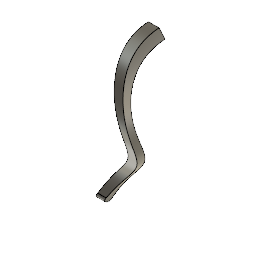
6.5 circular pattern (Autodesk Fusion 360 design; units mm, degrees)
Autodesk Fusion 360 part; units mm, degrees
sketch "Sketch1" plane through (0, 0, 0) normal (1, 0, 0) x (0, 1, 0)
  spline S0 degree 5 poles (0, 0) (-1.5461, -0.056) (-4.5103, -0.2863) (-8.5728, -0.9868) (-13.2055, -2.6049) (-17.6093, -5.6119) (-20.5447, -9.3915) (-21.9764, -13.7078) (-21.9581, -18.3281) (-20.7021, -23.054) (-18.5832, -27.735) (-16.0525, -32.2598) (-13.5801, -36.5535) (-11.5892, -40.5752) (-10.3932, -44.316) (-10.1254, -47.8001) (-10.6672, -50.4131) (-11.4827, -52.2914) (-12.2041, -53.5097) (-12.6092, -54.1104) knots 0 0 0 0 0 0 0.066667 0.133333 0.2 0.266667 0.333333 0.4 0.466667 0.533333 0.6 0.666667 0.733333 0.8 0.866667 0.933333 1 1 1 1 1 1
  line L0 (10.2739, 0.3719) -> (-10.2739, -0.3719)
  spline S1 degree 3 poles (0.1, -2.7622) (-6.0917, -2.9863) (-10.7245, -4.4824) (-13.8238, -6.6593) (-16.4227, -8.4848) (-17.9499, -10.7212) (-18.6267, -13.1732) (-19.304, -15.6268) (-19.1099, -18.3726) (-18.1871, -21.3366) (-17.1185, -24.7688) (-15.0764, -28.4198) (-13.0449, -32.0268) (-10.8363, -35.9482) (-8.7042, -39.8469) (-7.8006, -43.7909) (-7.1465, -46.6457) (-7.1496, -49.5409) (-7.9606, -52.2548) (-8.3548, -53.5742) (-8.9304, -54.8446) (-9.6679, -56.0549) knots 0 0 0 0 0.16767 0.16767 0.16767 0.30827 0.30827 0.30827 0.448963 0.448963 0.448963 0.611881 0.611881 0.611881 0.789001 0.789001 0.789001 0.917212 0.917212 0.917212 0.979548 0.979548 0.979548 0.979548
  line L1 (-12.2892, -55.9) -> (-11.545, -56.4354)
  line L2 (0, 0) -> (0.1, -2.7622)
  arc A0 (-12.6092, -54.1104) -> (-12.2892, -55.9) centre (-11.5269, -54.8403) ccw
  arc A1 (-11.545, -56.4354) -> (-9.6679, -56.0549) centre (-10.7827, -55.3757) ccw
  point P0 (-11.7402, -40.6199)
  dimension "d2" = 1.3054
  constraint coincident S0.start L2.start
  constraint midpoint S0.start L0
  constraint tangent S0 A0
  constraint tangent L1 A0
  constraint tangent L1 A1
  constraint tangent S1 A1
  constraint equal A0 A1
  measures "d2" radius of A0
sketch "Sketch2" plane through (0, 0, 0) normal (0, 1, 0) x (1, 0, 0)
  spline S0 degree 5 poles (-12.1026, -4.473) (-11.4157, -3.9229) (-10.0727, -2.8011) (-8.1507, -1.0537) (-5.7739, 1.4062) (-3.1241, 4.6972) (-0.8218, 8.197) (1.0858, 11.8869) (2.526, 15.7315) (3.3928, 19.6719) (3.574, 23.6369) (2.9838, 27.5566) (1.5945, 31.3748) (-0.5288, 35.0626) (-3.1973, 38.6306) (-6.1455, 42.1158) (-9.0701, 45.5713) (-11.6717, 49.0549) (-13.6924, 52.6195) (-14.9643, 56.3) (-15.3996, 60.1153) (-15.05, 63.2818) (-14.3933, 65.7216) (-13.7809, 67.3768) (-13.431, 68.2116) knots 0 0 0 0 0 0 0.05 0.1 0.15 0.2 0.25 0.3 0.35 0.4 0.45 0.5 0.55 0.6 0.65 0.7 0.75 0.8 0.85 0.9 0.95 1 1 1 1 1 1
  spline S1 degree 3 poles (-10.1736, -6.8817) (-5.8254, -3.3995) (-2.1215, 0.602) (0.7843, 5.1235) (3.2088, 8.8961) (5.0948, 13.0413) (5.978, 17.4473) (6.6428, 20.764) (6.6923, 24.2313) (5.9419, 27.5965) (5.2452, 30.7205) (3.8541, 33.7189) (2.0777, 36.4763) (-0.3869, 40.3021) (-3.5439, 43.7195) (-6.1481, 46.9634) (-8.2297, 49.5562) (-9.9166, 52.025) (-10.9152, 54.4302) (-12.1481, 57.3997) (-12.4388, 60.2799) (-11.7039, 63.5633) (-11.4557, 64.6723) (-11.0858, 65.8238) (-10.585, 67.0188) knots 0 0 0 0 0.179562 0.179562 0.179562 0.329386 0.329386 0.329386 0.442169 0.442169 0.442169 0.546866 0.546866 0.546866 0.692126 0.692126 0.692126 0.808235 0.808235 0.808235 0.951586 0.951586 0.951586 1 1 1 1
  line L0 (-10.1736, -6.8817) -> (-12.1026, -4.473)
  line L1 (-10.585, 67.0188) -> (-13.431, 68.2116)
  point P0 (1.1818, 12.4171)
  point P1 (1.5613, 31.0153)
  point P2 (-12.1026, 49.993)
  dimension "d8" = 3.0859
extrude "Extrude1" add sketch "Sketch2" along normal mid plane 90.686 makes body 1
extrude "Extrude2" add sketch "Sketch1" along normal mid plane 63.566 separate body makes body 2
combine "Combine1" operation intersect target body 1 tool bodies 2
